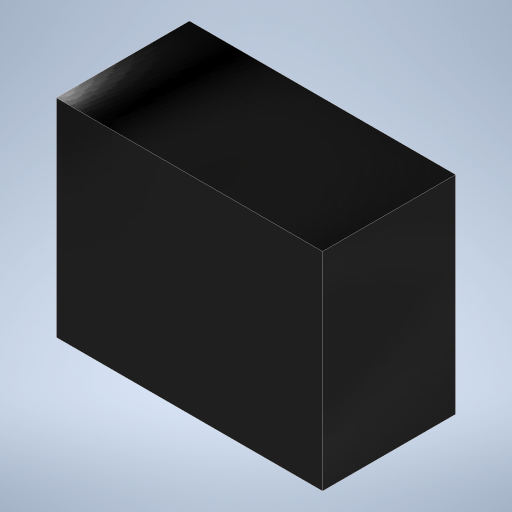
# Autodesk Inventor part: Sensor
Saved by Autodesk Inventor 2023 (Build 270158000, 158)
## iProperties
Created: 2023-01-17
Part Number: Sensor
Material: Generisch
Document SubType Name: Modeling
Designer: remoh
Density: 1 g/cm^3
Appearance: Schwarz
Author: remoh
Autodesk Inventor part; units mm, degrees
ref_plane "YZ Plane" through (0, 0, 0) normal (1, 0, 0) x (0, 1, 0)
ref_plane "XZ Plane" through (0, 0, 0) normal (0, 1, 0) x (-1, 0, 0)
ref_plane "XY Plane" through (0, 0, 0) normal (0, 0, 1) x (1, 0, 0)
sketch "Skizze1" plane through (0, 0, 0) normal (0, 0, 1) x (1, 0, 0)
  line L0 (0, 0) -> (3.4, 0)
  line L1 (3.4, 0) -> (3.4, -2.65)
  line L2 (3.4, -2.65) -> (0, -2.65)
  line L3 (0, -2.65) -> (0, 0)
  dimension "d0" = 2.65
  dimension "d1" = 3.4
  constraints: 8 end point, 2 parallel, 1 horizontal, 1 perpendicular
  measures "d0" distance of L2.end L0.start
  measures "d1" distance of L0.start L0.end
extrude "Extrusion1" add sketch "Skizze1" along normal blind 1.7
